Autodesk Inventor part; units mm, degrees
(part 2 of 2)
sketch "Sketch6" plane through (4.7625, 0, 0) normal (1, 0, 0) x (0, 0, -1)
  arc A0 (170.8837, 294.4565) -> (172.0866, 287.8113) centre (174.8077, 291.7353) ccw construction
  line L0 (170.8837, 294.4565) -> (172.7922, 297.2086) construction
  arc A1 (174.2704, 299.1942) -> (172.7922, 297.2086) centre (203.0571, 276.2209) ccw construction
  line L1 (174.2704, 299.1942) -> (186.7738, 314.8615) construction
  arc A2 (195.2416, 312.4978) -> (186.7738, 314.8615) centre (190.5061, 311.8829) ccw construction
  line L2 (195.2416, 312.4978) -> (195.6829, 309.0987) construction
  arc A3 (195.1019, 306.1294) -> (195.6829, 309.0987) centre (190.9475, 308.4838) ccw construction
  arc A4 (195.1019, 306.1294) -> (196.1286, 295.6536) centre (203.0571, 301.6209) ccw construction
  arc A5 (196.7071, 294.0954) -> (196.1286, 295.6536) centre (194.3195, 294.0954) ccw construction
  line L3 (196.7071, 294.0954) -> (196.7071, 292.4021) construction
  arc A6 (195.454, 290.3012) -> (196.7071, 292.4021) centre (194.3195, 292.4021) ccw construction
  arc A7 (195.454, 290.3012) -> (188.9768, 283.824) centre (203.0571, 276.2209) ccw construction
  arc A8 (186.8759, 282.5709) -> (188.9768, 283.824) centre (186.8759, 284.9585) ccw construction
  line L4 (186.8759, 282.5709) -> (186.0222, 282.5709) construction
  arc A9 (183.1524, 283.5294) -> (186.0222, 282.5709) centre (186.0222, 287.3461) ccw construction
  arc A10 (183.1524, 283.5294) -> (177.3062, 285.3581) centre (177.6571, 276.2209) ccw construction
  arc A11 (174.4018, 286.2058) -> (177.3062, 285.3581) centre (177.1229, 290.1298) ccw construction
  line L5 (174.4018, 286.2058) -> (172.0866, 287.8113) construction
  arc A12 (298.3468, 346.8044) -> (302.3019, 353.3428) centre (297.8735, 351.556) ccw construction
  line L6 (298.3468, 346.8044) -> (283.1869, 345.2944) construction
  arc A13 (278.6486, 347.5403) -> (283.1869, 345.2944) centre (282.7136, 350.046) ccw construction
  arc A14 (278.6486, 347.5403) -> (268.2318, 356.07) centre (261.0807, 336.7111) ccw construction
  arc A15 (265.1348, 360.076) -> (268.2318, 356.07) centre (269.8865, 360.5493) ccw construction
  line L7 (265.1348, 360.076) -> (263.6248, 375.236) construction
  arc A16 (269.2547, 380.403) -> (263.6248, 375.236) centre (268.3765, 375.7093) ccw construction
  arc A17 (302.3019, 353.3428) -> (269.2547, 380.403) centre (261.0807, 336.7111) ccw construction
  arc A18 (379.8681, 143.7131) -> (386.4173, 137.5565) centre (384.2479, 141.8105) ccw construction
  line L8 (379.8681, 143.7131) -> (390.24, 167.5887) construction
  arc A19 (394.413, 170.4568) -> (390.24, 167.5887) centre (394.6197, 165.686) ccw construction
  arc A20 (394.413, 170.4568) -> (413.0231, 184.3286) centre (393.5194, 191.0749) ccw construction
  arc A21 (416.9638, 187.5084) -> (413.0231, 184.3286) centre (417.536, 182.7676) ccw construction
  line L9 (416.9638, 187.5084) -> (432.089, 189.3339) construction
  arc A22 (437.3722, 183.813) -> (432.089, 189.3339) centre (432.6612, 184.5931) ccw construction
  arc A23 (413.7134, 151.4769) -> (437.3722, 183.813) centre (393.5194, 191.0749) ccw construction
  line L10 (413.7134, 151.4769) -> (386.4173, 137.5565) construction
  arc A24 (430.5672, 201.9424) -> (434.3852, 208.5618) centre (429.995, 206.6832) ccw construction
  line L11 (430.5672, 201.9424) -> (415.442, 200.1169) construction
  arc A25 (410.858, 202.2678) -> (415.442, 200.1169) centre (414.8698, 204.8577) ccw construction
  arc A26 (410.858, 202.2678) -> (400.2657, 210.5786) centre (393.5194, 191.0749) ccw construction
  arc A27 (397.0859, 214.5193) -> (400.2657, 210.5786) centre (401.8267, 215.0914) ccw construction
  line L12 (397.0859, 214.5193) -> (395.2604, 229.6445) construction
  arc A28 (400.7814, 234.9277) -> (395.2604, 229.6445) centre (400.0012, 230.2167) ccw construction
  arc A29 (434.3852, 208.5618) -> (400.7814, 234.9277) centre (393.5194, 191.0749) ccw construction
  arc A30 (250.9874, 373.9773) -> (244.449, 377.9323) centre (246.2357, 373.504) ccw construction
  line L13 (250.9874, 373.9773) -> (252.4974, 358.8173) construction
  arc A31 (250.2514, 354.2791) -> (252.4974, 358.8173) centre (247.7457, 358.344) ccw construction
  arc A32 (250.2514, 354.2791) -> (241.7218, 343.8623) centre (261.0807, 336.7111) ccw construction
  arc A33 (237.7157, 340.7653) -> (241.7218, 343.8623) centre (237.2424, 345.5169) ccw construction
  line L14 (237.7157, 340.7653) -> (216.1032, 338.6126) construction
  arc A34 (211.8976, 346.3429) -> (216.1032, 338.6126) centre (215.6299, 343.3643) ccw construction
  line L15 (211.8976, 346.3429) -> (226.3381, 364.4375) construction
  arc A35 (244.449, 377.9323) -> (226.3381, 364.4375) centre (261.0807, 336.7111) ccw construction
  arc A36 (198.999, 204.1865) -> (205.9543, 209.4304) centre (201.2979, 208.3719) ccw construction
  line L16 (198.999, 204.1865) -> (188.5021, 209.9521) construction
  arc A37 (186.0315, 214.3721) -> (188.5021, 209.9521) centre (190.801, 214.1375) ccw construction
  arc A38 (186.0315, 214.3721) -> (185.1217, 221.5267) centre (165.4189, 215.3861) ccw construction
  arc A39 (186.4073, 226.4244) -> (185.1217, 221.5267) centre (189.6806, 222.9476) ccw construction
  line L17 (186.4073, 226.4244) -> (193.2473, 232.864) construction
  arc A40 (201.177, 230.4457) -> (193.2473, 232.864) centre (196.5206, 229.3871) ccw construction
  line L18 (201.177, 230.4457) -> (205.9543, 209.4304) construction
  arc A41 (211.3352, 325.3748) -> (207.073, 320.0083) centre (211.8085, 320.6231) ccw construction
  line L19 (211.3352, 325.3748) -> (238.9744, 328.1278) construction
  arc A42 (243.5127, 325.8818) -> (238.9744, 328.1278) centre (239.4477, 323.3761) ccw construction
  arc A43 (243.5127, 325.8818) -> (244.321, 324.6686) centre (261.0807, 336.7111) ccw construction
  arc A44 (244.646, 319.6154) -> (244.321, 324.6686) centre (240.4431, 321.8822) ccw construction
  line L20 (244.646, 319.6154) -> (226.8389, 286.5977) construction
  arc A45 (224.633, 284.5268) -> (226.8389, 286.5977) centre (222.636, 288.8644) ccw construction
  arc A46 (224.633, 284.5268) -> (222.4898, 283.1494) centre (228.4571, 276.2209) ccw construction
  arc A47 (220.9317, 282.5709) -> (222.4898, 283.1494) centre (220.9317, 284.9585) ccw construction
  line L21 (220.9317, 282.5709) -> (219.2384, 282.5709) construction
  arc A48 (217.1375, 283.824) -> (219.2384, 282.5709) centre (219.2384, 284.9585) ccw construction
  arc A49 (217.1375, 283.824) -> (210.6603, 290.3012) centre (203.0571, 276.2209) ccw construction
  arc A50 (209.4071, 292.4021) -> (210.6603, 290.3012) centre (211.7947, 292.4021) ccw construction
  line L22 (209.4071, 292.4021) -> (209.4071, 294.0954) construction
  arc A51 (209.9856, 295.6536) -> (209.4071, 294.0954) centre (211.7947, 294.0954) ccw construction
  arc A52 (209.9856, 295.6536) -> (209.5973, 308.0115) centre (203.0571, 301.6209) ccw construction
  arc A53 (208.2772, 310.7339) -> (209.5973, 308.0115) centre (213.0127, 311.3488) ccw construction
  line L23 (208.2772, 310.7339) -> (207.073, 320.0083) construction
  arc A54 (219.2384, 269.8709) -> (217.1375, 268.6177) centre (219.2384, 267.4833) ccw construction
  line L24 (219.2384, 269.8709) -> (220.9317, 269.8709) construction
  arc A55 (222.4898, 269.2924) -> (220.9317, 269.8709) centre (220.9317, 267.4833) ccw construction
  arc A56 (222.4898, 269.2924) -> (232.2342, 267.8934) centre (228.4571, 276.2209) ccw construction
  arc A57 (235.2436, 268.2059) -> (232.2342, 267.8934) centre (234.2067, 263.5446) ccw construction
  line L25 (235.2436, 268.2059) -> (318.0387, 249.787) construction
  arc A58 (321.7764, 245.0563) -> (318.0387, 249.787) centre (317.0017, 245.1258) ccw construction
  line L26 (321.7764, 245.0563) -> (320.5418, 160.2462) construction
  arc A59 (319.5416, 157.3907) -> (320.5418, 160.2462) centre (315.7671, 160.3157) ccw construction
  arc A60 (319.5416, 157.3907) -> (317.8734, 149.6741) centre (326.7693, 151.7896) ccw construction
  arc A61 (317.6048, 146.6604) -> (317.8734, 149.6741) centre (313.2278, 148.5693) ccw construction
  line L27 (317.6048, 146.6604) -> (317.2174, 145.7719) construction
  arc A62 (315.236, 144.3478) -> (317.2174, 145.7719) centre (315.0288, 146.7264) ccw construction
  arc A63 (315.236, 144.3478) -> (306.8489, 141.0546) centre (316.6157, 128.5073) ccw construction
  arc A64 (304.4279, 140.7502) -> (306.8489, 141.0546) centre (305.3824, 142.9387) ccw construction
  line L28 (304.4279, 140.7502) -> (302.7698, 141.4733) construction
  arc A65 (301.5729, 142.6264) -> (302.7698, 141.4733) centre (303.7243, 143.6618) ccw construction
  arc A66 (301.5729, 142.6264) -> (291.2986, 147.5757) centre (293.3334, 138.661) ccw construction
  arc A67 (288.2875, 147.8716) -> (291.2986, 147.5757) centre (290.2359, 152.2312) ccw construction
  line L29 (288.2875, 147.8716) -> (248.8959, 165.4772) construction
  arc A68 (246.7674, 167.3507) -> (248.8959, 165.4772) centre (250.8444, 169.8368) ccw construction
  arc A69 (246.7674, 167.3507) -> (245.8371, 168.6073) centre (239.3128, 162.8049) ccw construction
  arc A70 (244.6507, 171.3375) -> (245.8371, 168.6073) centre (249.4053, 171.7808) ccw construction
  arc A71 (244.6507, 171.3375) -> (242.4292, 176.382) centre (235.9761, 170.5287) ccw construction
  line L30 (242.4292, 176.382) -> (231.9513, 187.9335) construction
  arc A72 (231.9513, 187.9335) -> (227.1533, 190.6337) centre (225.4982, 182.0802) ccw construction
  arc A73 (224.5561, 192.0782) -> (227.1533, 190.6337) centre (228.0605, 195.3219) ccw construction
  arc A74 (224.5561, 192.0782) -> (223.7494, 192.8453) centre (218.1439, 186.1428) ccw construction
  arc A75 (222.1565, 195.4498) -> (223.7494, 192.8453) centre (226.8129, 196.5083) ccw construction
  line L31 (222.1565, 195.4498) -> (211.1035, 244.0716) construction
  arc A76 (211.402, 247.0824) -> (211.1035, 244.0716) centre (215.7599, 245.1301) ccw construction
  arc A77 (211.402, 247.0824) -> (209.9856, 256.7882) centre (203.0571, 250.8209) ccw construction
  arc A78 (209.4071, 258.3463) -> (209.9856, 256.7882) centre (211.7947, 258.3463) ccw construction
  line L32 (209.4071, 258.3463) -> (209.4071, 260.0397) construction
  arc A79 (210.6603, 262.1405) -> (209.4071, 260.0397) centre (211.7947, 260.0397) ccw construction
  arc A80 (210.6603, 262.1405) -> (217.1375, 268.6177) centre (203.0571, 276.2209) ccw construction
  arc A81 (337.1993, 150.5599) -> (335.2123, 148.2783) centre (339.6214, 146.4446) ccw construction
  line L33 (337.1993, 150.5599) -> (367.2672, 168.2562) construction
  arc A82 (374.069, 162.2382) -> (367.2672, 168.2562) centre (369.6893, 164.1408) ccw construction
  line L34 (374.069, 162.2382) -> (363.4789, 137.8602) construction
  arc A83 (361.2833, 135.5164) -> (363.4789, 137.8602) centre (359.0991, 139.7628) ccw construction
  arc A84 (361.2833, 135.5164) -> (357.5507, 132.0949) centre (365.675, 126.9785) ccw construction
  arc A85 (355.0252, 130.1112) -> (357.5507, 132.0949) centre (353.51, 134.6396) ccw construction
  line L35 (355.0252, 130.1112) -> (345.8158, 127.0298) construction
  arc A86 (342.7902, 127.0282) -> (345.8158, 127.0298) centre (344.3006, 131.5582) ccw construction
  arc A87 (342.7902, 127.0282) -> (337.1978, 127.0899) centre (339.8979, 118.3537) ccw construction
  arc A88 (335.5383, 127.1825) -> (337.1978, 127.0899) centre (336.4928, 129.3711) ccw construction
  line L36 (335.5383, 127.1825) -> (335.1284, 127.3613) construction
  arc A89 (332.3207, 130.9922) -> (335.1284, 127.3613) centre (337.0372, 131.7384) ccw construction
  arc A90 (332.3207, 130.9922) -> (329.1629, 138.2741) centre (316.6157, 128.5073) ccw construction
  arc A91 (328.8585, 140.6951) -> (329.1629, 138.2741) centre (331.047, 139.7406) ccw construction
  line L37 (328.8585, 140.6951) -> (329.246, 141.5836) construction
  arc A92 (331.2718, 143.8309) -> (329.246, 141.5836) centre (333.623, 139.6747) ccw construction
  arc A93 (331.2718, 143.8309) -> (335.2123, 148.2783) centre (326.7693, 151.7896) ccw construction
  arc A94 (382.3265, 208.4134) -> (384.4774, 212.9975) centre (379.7366, 212.4253) ccw construction
  arc A95 (382.3265, 208.4134) -> (372.946, 189.4499) centre (393.5194, 191.0749) ccw construction
  arc A96 (370.6077, 184.9585) -> (372.946, 189.4499) centre (368.1856, 189.0739) ccw construction
  line L38 (370.6077, 184.9585) -> (340.6035, 167.2997) construction
  arc A97 (333.4067, 171.4846) -> (340.6035, 167.2997) centre (338.1814, 171.4151) ccw construction
  line L39 (333.4067, 171.4846) -> (334.4104, 240.4277) construction
  arc A98 (341.5331, 244.5162) -> (334.4104, 240.4277) centre (339.1851, 240.3582) ccw construction
  arc A99 (341.5331, 244.5162) -> (377.7123, 234.6667) centre (379.0508, 310.9542) ccw construction
  arc A100 (382.3693, 230.4644) -> (377.7123, 234.6667) centre (377.6285, 229.8922) ccw construction
  line L40 (382.3693, 230.4644) -> (384.4774, 212.9975) construction
  arc A101 (241.0284, 286.1531) -> (244.1944, 279.2252) centre (245.2313, 283.8864) ccw construction
  line L41 (241.0284, 286.1531) -> (255.824, 313.5869) construction
  arc A102 (260.2249, 316.0913) -> (255.824, 313.5869) centre (260.0269, 311.3202) ccw construction
  arc A103 (260.2249, 316.0913) -> (280.4395, 329.5599) centre (261.0807, 336.7111) ccw construction
  arc A104 (284.4456, 332.6569) -> (280.4395, 329.5599) centre (284.9189, 327.9052) ccw construction
  line L42 (284.4456, 332.6569) -> (299.6056, 334.1669) construction
  arc A105 (304.7726, 328.5371) -> (299.6056, 334.1669) centre (300.0789, 329.4152) ccw construction
  arc A106 (304.5076, 327.2295) -> (304.7726, 328.5371) centre (261.0807, 336.7111) ccw construction
  arc A107 (304.5076, 327.2295) -> (313.4045, 272.0681) centre (379.0508, 310.9542) ccw construction
  arc A108 (308.259, 264.9731) -> (313.4045, 272.0681) centre (309.296, 269.6344) ccw construction
  line L43 (308.259, 264.9731) -> (244.1944, 279.2252) construction
  arc A109 (185.1826, 269.8709) -> (183.6244, 269.2924) centre (185.1826, 267.4833) ccw construction
  line L44 (185.1826, 269.8709) -> (185.5094, 269.8709) construction
  arc A110 (189.5424, 267.6526) -> (185.5094, 269.8709) centre (185.5094, 265.0957) ccw construction
  arc A111 (189.5424, 267.6526) -> (195.454, 262.1405) centre (203.0571, 276.2209) ccw construction
  arc A112 (196.7071, 260.0397) -> (195.454, 262.1405) centre (194.3195, 260.0397) ccw construction
  line L45 (196.7071, 260.0397) -> (196.7071, 259.1859) construction
  arc A113 (195.7486, 256.3162) -> (196.7071, 259.1859) centre (191.9319, 259.1859) ccw construction
  arc A114 (195.7486, 256.3162) -> (194.0462, 252.3753) centre (203.0571, 250.8209) ccw construction
  arc A115 (192.6138, 249.7103) -> (194.0462, 252.3753) centre (189.3405, 253.1871) ccw construction
  line L46 (192.6138, 249.7103) -> (177.7018, 235.6713) construction
  arc A116 (172.7356, 234.683) -> (177.7018, 235.6713) centre (174.4285, 239.1481) ccw construction
  arc A117 (172.7356, 234.683) -> (164.402, 235.9985) centre (165.4189, 215.3861) ccw construction
  arc A118 (159.9817, 238.4684) -> (164.402, 235.9985) centre (164.1668, 240.7679) ccw construction
  line L47 (159.9817, 238.4684) -> (154.2435, 248.9118) construction
  arc A119 (155.9126, 255.2699) -> (154.2435, 248.9118) centre (158.4286, 251.2113) ccw construction
  line L48 (155.9126, 255.2699) -> (173.8931, 266.4164) construction
  arc A120 (176.8373, 267.1137) -> (173.8931, 266.4164) centre (176.4091, 262.3577) ccw construction
  arc A121 (176.8373, 267.1137) -> (183.6244, 269.2924) centre (177.6571, 276.2209) ccw construction
  circle A122 centre (62.0508, 103.0707) radius 3.2512 construction
  circle A123 centre (365.675, 126.9785) radius 3.2512 construction
  circle A124 centre (116.952, 9.0853) radius 3.2512 construction
  circle A125 centre (143.5951, 255.1053) radius 3.2512 construction
  circle A126 centre (199.3, 330.5575) radius 3.2512 construction
  circle A127 centre (219.5153, 55.5753) radius 3.2512 construction
  line L49 (167.5741, 300.8271) -> (63.5783, 150.8617) construction
  arc A128 (63.5783, 150.8617) -> (59.1713, 138.8602) centre (84.4507, 136.3874) ccw construction
  line L50 (59.1713, 138.8602) -> (51.0413, 55.7455) construction
  arc A129 (51.0413, 55.7455) -> (122.6227, 4.5541) centre (101.6, 50.8) ccw construction
  line L51 (122.6227, 4.5541) -> (278.1353, 75.2478) construction
  arc A130 (278.1353, 75.2478) -> (279.5746, 75.9415) centre (263.4194, 107.6199) ccw construction
  line L52 (279.5746, 75.9415) -> (416.5983, 145.82) construction
  arc A131 (416.5983, 145.82) -> (387.4324, 241.5089) centre (393.5194, 191.0749) ccw construction
  arc A132 (310.7115, 325.875) -> (387.4324, 241.5089) centre (379.0508, 310.9542) ccw construction
  arc A133 (310.7115, 325.875) -> (221.3748, 368.3984) centre (261.0807, 336.7111) ccw construction
  line L53 (221.3748, 368.3984) -> (169.3072, 303.1551) construction
  arc A134 (169.3072, 303.1551) -> (167.5741, 300.8271) centre (203.0571, 276.2209) ccw construction
  circle A135 centre (326.7693, 151.7896) radius 2.794 construction
  circle A136 centre (172.549, 123.5241) radius 3.2512 construction
  circle A137 centre (203.0571, 276.2209) radius 9.652 construction
  circle A138 centre (228.4571, 276.2209) radius 2.794 construction
  circle A139 centre (203.0571, 250.8209) radius 2.794 construction
  circle A140 centre (177.6571, 276.2209) radius 2.794 construction
  circle A141 centre (84.4507, 136.3874) radius 14.2875 construction
  circle A142 centre (263.4194, 107.6199) radius 14.2875 construction
  circle A143 centre (316.6157, 128.5073) radius 9.5504 construction
  circle A144 centre (239.3128, 162.8049) radius 2.3812 construction
  circle A145 centre (218.1439, 186.1428) radius 2.3876 construction
  arc A146 (219.8851, 180.1779) -> (219.7225, 176.8412) centre (221.4722, 178.4283) ccw construction
  line L54 (219.8851, 180.1779) -> (223.9112, 183.8298) construction
  arc A147 (227.2479, 183.6672) -> (223.9112, 183.8298) centre (225.4982, 182.0802) ccw construction
  line L55 (227.2479, 183.6672) -> (237.7258, 172.1157) construction
  arc A148 (237.5632, 168.779) -> (237.7258, 172.1157) centre (235.9761, 170.5287) ccw construction
  line L56 (237.5632, 168.779) -> (233.5371, 165.1271) construction
  arc A149 (230.2004, 165.2897) -> (233.5371, 165.1271) centre (231.9501, 166.8768) ccw construction
  line L57 (230.2004, 165.2897) -> (219.7225, 176.8412) construction
  circle A150 centre (339.8979, 118.3537) radius 2.794 construction
  circle A151 centre (306.462, 105.2251) radius 2.794 construction
  circle A152 centre (293.3334, 138.661) radius 2.794 construction
  circle A153 centre (103.7307, 197.6195) radius 3.2512 construction
  circle A154 centre (203.0571, 301.6209) radius 2.794 construction
  circle A155 centre (101.6, 50.8) radius 14.2875 construction
  circle A156 centre (165.4189, 215.3861) radius 14.2875 construction
  circle A157 centre (393.5194, 191.0749) radius 14.2875 construction
  circle A158 centre (261.0807, 336.7111) radius 14.2875 construction
  line L58 (68.7964, 147.2431) -> (172.7922, 297.2086) construction
  arc A159 (174.2704, 299.1942) -> (172.7922, 297.2086) centre (203.0571, 276.2209) ccw construction
  line L59 (174.2704, 299.1942) -> (226.3381, 364.4375) construction
  arc A160 (304.5076, 327.2295) -> (226.3381, 364.4375) centre (261.0807, 336.7111) ccw construction
  arc A161 (304.5076, 327.2295) -> (388.1933, 235.2047) centre (379.0508, 310.9542) ccw construction
  arc A162 (413.7134, 151.4769) -> (388.1933, 235.2047) centre (393.5194, 191.0749) ccw construction
  line L60 (413.7134, 151.4769) -> (276.6898, 81.5983) construction
  arc A163 (275.5075, 81.0285) -> (276.6898, 81.5983) centre (263.4194, 107.6199) ccw construction
  line L61 (275.5075, 81.0285) -> (119.9949, 10.3348) construction
  arc A164 (57.3611, 55.1273) -> (119.9949, 10.3348) centre (101.6, 50.8) ccw construction
  line L62 (57.3611, 55.1273) -> (65.4912, 138.242) construction
  arc A165 (68.7964, 147.2431) -> (65.4912, 138.242) centre (84.4507, 136.3874) ccw construction
  circle A166 centre (143.5951, 255.1053) radius 9.6012 construction
  circle A167 centre (165.4189, 215.3861) radius 20.6375 construction
  circle A168 centre (103.7307, 197.6195) radius 9.6012 construction
  circle A169 centre (172.549, 123.5241) radius 9.6012 construction
  circle A170 centre (84.4507, 136.3874) radius 20.6375 construction
  circle A171 centre (62.0508, 103.0707) radius 9.6012 construction
  circle A172 centre (218.1439, 186.1428) radius 8.7376 construction
  arc A173 (215.6189, 184.8813) -> (215.0191, 172.575) centre (221.4722, 178.4283) ccw construction
  line L63 (215.6189, 184.8813) -> (219.6449, 188.5332) construction
  arc A174 (231.9513, 187.9335) -> (219.6449, 188.5332) centre (225.4982, 182.0802) ccw construction
  line L64 (231.9513, 187.9335) -> (242.4292, 176.382) construction
  arc A175 (241.8294, 164.0757) -> (242.4292, 176.382) centre (235.9761, 170.5287) ccw construction
  line L65 (241.8294, 164.0757) -> (237.8033, 160.4238) construction
  arc A176 (225.497, 161.0235) -> (237.8033, 160.4238) centre (231.9501, 166.8768) ccw construction
  line L66 (225.497, 161.0235) -> (215.0191, 172.575) construction
  circle A177 centre (239.3128, 162.8049) radius 8.7312 construction
  circle A178 centre (293.3334, 138.661) radius 9.144 construction
  circle A179 centre (316.6157, 128.5073) radius 15.9004 construction
  circle A180 centre (306.462, 105.2251) radius 9.144 construction
  circle A181 centre (263.4194, 107.6199) radius 20.6375 construction
  circle A182 centre (219.5153, 55.5753) radius 9.6012 construction
  circle A183 centre (101.6, 50.8) radius 20.6375 construction
  circle A184 centre (116.952, 9.0853) radius 9.6012 construction
  line L67 (145.5875, 209.6745) -> (112.9569, 200.2767) construction
  line L68 (148.2185, 246.6906) -> (155.4809, 233.4731) construction
  line L69 (167.016, 194.8105) -> (171.806, 133.0965) construction
  line L70 (100.8472, 188.4616) -> (90.6488, 156.0722) construction
  line L71 (104.8717, 133.4057) -> (163.0486, 124.9113) construction
  line L72 (183.4664, 205.3763) -> (210.5028, 190.3808) construction
  line L73 (179.6605, 129.9747) -> (220.2581, 166.7992) construction
  line L74 (242.808, 154.8037) -> (255.1581, 126.5317) construction
  line L75 (247.2842, 159.2422) -> (284.9853, 142.3921) construction
  line L76 (286.9883, 132.0768) -> (277.7401, 122.4801) construction
  line L77 (284.0251, 106.4735) -> (297.3321, 105.7331) construction
  line L78 (310.2595, 113.9327) -> (310.1173, 113.6067) construction
  line L79 (301.715, 135.0057) -> (302.041, 134.8635) construction
  line L80 (250.1124, 91.8456) -> (225.7061, 62.914) construction
  line L81 (243.091, 111.1778) -> (182.0065, 121.8689) construction
  line L82 (178.0082, 115.626) -> (214.0561, 63.4734) construction
  line L83 (165.8443, 116.6517) -> (116.0115, 65.5721) construction
  line L84 (122.2206, 51.6351) -> (209.922, 55.1868) construction
  line L85 (108.7277, 31.4324) -> (113.6359, 18.0956) construction
  line L86 (87.1885, 36.0279) -> (70.5598, 18.9832) construction
  line L87 (88.5053, 116.1521) -> (97.5454, 71.0353) construction
  line L88 (67.8439, 95.4142) -> (89.1479, 67.2575) construction
  line L89 (72.936, 119.2609) -> (67.4078, 111.0385) construction
  line L90 (142.4146, 244.0672) -> (148.8512, 232.3527)
  line L91 (141.7059, 215.1647) -> (122.3457, 209.5888)
  arc A185 (139.8047, 246.284) -> (140.0117, 246.1979) centre (143.5951, 255.1053) ccw
  arc A186 (148.5657, 227.2972) -> (145.0885, 218.9327) centre (165.4189, 215.3861) ccw
  line L92 (117.1001, 216.8987) -> (136.9001, 245.4509)
  arc A187 (148.5657, 227.2972) -> (148.8512, 232.3527) centre (144.6661, 230.0532) ccw
  arc A188 (141.7059, 215.1647) -> (145.0885, 218.9327) centre (140.3843, 219.7534) ccw
  arc A189 (142.4146, 244.0672) -> (140.0117, 246.1979) centre (138.2295, 241.7677) ccw
  arc A190 (117.1001, 216.8987) -> (122.3457, 209.5888) centre (121.0241, 214.1775) ccw
  circle A191 centre (138.8621, 244.0903) radius 2.3876 construction
  arc A192 (139.8047, 246.284) -> (136.9001, 245.4509) centre (138.8621, 244.0903) ccw
  line L93 (145.2207, 202.9608) -> (114.238, 194.0376)
  line L94 (107.0529, 187.0272) -> (97.3696, 156.2736)
  line L95 (107.9765, 139.3697) -> (159.6899, 131.819)
  line L96 (160.8561, 192.1151) -> (165.1407, 136.9136)
  arc A193 (104.1161, 142.6465) -> (98.6409, 151.3722) centre (84.4507, 136.3874) ccw
  arc A194 (150.0893, 201.5691) -> (157.8472, 196.1878) centre (165.4189, 215.3861) ccw
  arc A195 (108.9913, 189.5877) -> (111.6305, 192.1628) centre (103.7307, 197.6195) ccw
  arc A196 (97.3696, 156.2736) -> (98.6409, 151.3722) centre (101.9243, 154.8395) ccw
  arc A197 (104.1161, 142.6465) -> (107.9765, 139.3697) centre (108.6664, 144.0948) ccw
  arc A198 (159.6899, 131.819) -> (165.1407, 136.9136) centre (160.3798, 136.5441) ccw
  arc A199 (150.0893, 201.5691) -> (145.2207, 202.9608) centre (146.5423, 198.3721) ccw
  arc A200 (160.8561, 192.1151) -> (157.8472, 196.1878) centre (156.0952, 191.7456) ccw
  arc A201 (114.238, 194.0376) -> (111.6305, 192.1628) centre (115.5595, 189.4489) ccw
  arc A202 (108.9913, 189.5877) -> (107.0529, 187.0272) centre (111.6076, 185.5931) ccw
  line L97 (182.3196, 198.751) -> (208.3567, 184.3098)
  line L98 (173.518, 193.0979) -> (177.1237, 146.6426)
  line L99 (185.0928, 143.4752) -> (212.7408, 168.5537)
  arc A203 (175.8624, 197.5861) -> (177.263, 198.4856) centre (165.4189, 215.3861) ccw
  arc A204 (210.3177, 182.2574) -> (211.6131, 180.3381) centre (218.1439, 186.1428) ccw
  arc A205 (212.7982, 177.6127) -> (213.775, 174.2825) centre (221.8723, 178.4659) ccw
  arc A206 (177.1237, 146.6426) -> (185.0928, 143.4752) centre (181.8846, 147.0122) ccw
  arc A207 (182.3196, 198.751) -> (177.263, 198.4856) centre (180.0035, 194.5751) ccw
  arc A208 (175.8624, 197.5861) -> (173.518, 193.0979) centre (178.2789, 193.4674) ccw
  arc A209 (212.7408, 168.5537) -> (213.775, 174.2825) centre (209.5326, 172.0906) ccw
  arc A210 (212.7982, 177.6127) -> (211.6131, 180.3381) centre (208.044, 177.1657) ccw
  arc A211 (210.3177, 182.2574) -> (208.3567, 184.3098) centre (206.0406, 180.1339) ccw
  line L100 (193.6591, 134.0992) -> (221.2962, 159.1677)
  line L101 (236.5596, 153.2447) -> (248.4542, 126.0155)
  line L102 (242.0082, 117.8138) -> (196.0441, 125.8585)
  arc A212 (247.7126, 121.0065) -> (246.7001, 119.7182) centre (263.4194, 107.6199) ccw
  arc A213 (232.9035, 156.8757) -> (234.7042, 155.389) centre (239.3128, 162.8049) ccw
  arc A214 (227.1405, 159.6124) -> (230.3016, 158.322) centre (231.9501, 166.8768) ccw
  line L103 (224.5243, 162.0959) -> (225.497, 161.0235)
  arc A215 (193.6591, 134.0992) -> (196.0441, 125.8585) centre (196.8673, 130.5622) ccw
  arc A216 (247.7126, 121.0065) -> (248.4542, 126.0155) centre (244.0783, 124.104) ccw
  arc A217 (242.0082, 117.8138) -> (246.7001, 119.7182) centre (242.8314, 122.5175) ccw
  arc A218 (227.1405, 159.6124) -> (221.2962, 159.1677) centre (224.5044, 155.6308) ccw
  arc A219 (232.9035, 156.8757) -> (230.3016, 158.322) centre (229.3981, 153.633) ccw
  arc A220 (236.5596, 153.2447) -> (234.7042, 155.389) centre (232.1837, 151.3332) ccw
  line L104 (303.8285, 115.0715) -> (303.9854, 115.4311)
  line L105 (297.693, 129.8322) -> (298.103, 129.6534)
  line L106 (292.1012, 128.2313) -> (284.8365, 120.693)
  line L107 (288.0097, 112.6116) -> (298.4626, 112.03)
  arc A221 (283.3782, 112.8693) -> (281.6177, 117.3529) centre (263.4194, 107.6199) ccw
  arc A222 (301.9596, 113.1838) -> (301.3812, 112.8276) centre (306.462, 105.2251) ccw
  arc A223 (294.7827, 129.6326) -> (296.0335, 129.9248) centre (293.3334, 138.661) ccw
  arc A224 (300.9106, 126.0225) -> (303.4157, 119.6426) centre (316.6157, 128.5073) ccw
  arc A225 (300.9106, 126.0225) -> (298.103, 129.6534) centre (296.1941, 125.2763) ccw
  arc A226 (303.8285, 115.0715) -> (303.4157, 119.6426) centre (299.4515, 116.9804) ccw
  arc A227 (301.9596, 113.1838) -> (303.9854, 115.4311) centre (299.6083, 117.34) ccw
  arc A228 (298.4626, 112.03) -> (301.3812, 112.8276) centre (298.7279, 116.7978) ccw
  arc A229 (284.8365, 120.693) -> (288.0097, 112.6116) centre (288.275, 117.3794) ccw
  arc A230 (294.7827, 129.6326) -> (292.1012, 128.2313) centre (295.5396, 124.9178) ccw
  circle A231 centre (296.7386, 127.6436) radius 2.3876 construction
  arc A232 (297.693, 129.8322) -> (296.0335, 129.9248) centre (296.7386, 127.6436) ccw
  line L108 (262.9615, 145.28) -> (276.2747, 139.3298)
  line L109 (277.7647, 131.6567) -> (274.7017, 128.4782)
  line L110 (256.6371, 139.0089) -> (260.0922, 131.0994)
  arc A233 (269.7893, 127.2498) -> (264.2711, 128.2398) centre (263.4194, 107.6199) ccw
  arc A234 (262.9615, 145.28) -> (256.6371, 139.0089) centre (261.013, 140.9204) ccw
  arc A235 (277.7647, 131.6567) -> (276.2747, 139.3298) centre (274.3263, 134.9702) ccw
  arc A236 (269.7893, 127.2498) -> (274.7017, 128.4782) centre (271.2632, 131.7918) ccw
  arc A237 (260.0922, 131.0994) -> (264.2711, 128.2398) centre (264.4682, 133.011) ccw
  line L111 (285.8795, 100.0105) -> (292.479, 99.6433)
  line L112 (253.5407, 86.0614) -> (246.6512, 77.8946)
  line L113 (252.2773, 70.4684) -> (275.5075, 81.0285)
  line L114 (294.3831, 90.6215) -> (276.6898, 81.5983)
  arc A238 (275.5075, 81.0285) -> (276.6898, 81.5983) centre (263.4194, 107.6199) ccw
  arc A239 (258.3611, 87.6119) -> (281.4437, 97.5684) centre (263.4194, 107.6199) ccw
  arc A240 (258.3611, 87.6119) -> (253.5407, 86.0614) centre (257.1906, 82.9824) ccw
  arc A241 (246.6512, 77.8946) -> (252.2773, 70.4684) centre (250.3012, 74.8155) ccw
  arc A242 (285.8795, 100.0105) -> (281.4437, 97.5684) centre (285.6142, 95.2426) ccw
  arc A243 (299.5399, 99.2504) -> (305.2476, 96.1621) centre (306.462, 105.2251) ccw
  arc A244 (294.3831, 90.6215) -> (292.479, 99.6433) centre (292.2137, 94.8754) ccw
  line L115 (239.8187, 105.304) -> (197.6387, 112.6864)
  line L116 (192.8872, 105.2675) -> (216.4656, 71.1553)
  line L117 (243.8334, 94.2504) -> (224.0438, 70.7914)
  arc A245 (243.5849, 101.9193) -> (244.5496, 99.2631) centre (263.4194, 107.6199) ccw
  arc A246 (197.6387, 112.6864) -> (192.8872, 105.2675) centre (196.8154, 107.9827) ccw
  arc A247 (243.5849, 101.9193) -> (239.8187, 105.304) centre (238.9955, 100.6003) ccw
  arc A248 (243.8334, 94.2504) -> (244.5496, 99.2631) centre (240.1835, 97.3294) ccw
  arc A249 (216.4656, 71.1553) -> (224.0438, 70.7914) centre (220.3938, 73.8705) ccw
  line L118 (106.1416, 126.803) -> (150.0332, 120.3943)
  line L119 (95.1658, 115.2322) -> (103.3374, 74.4504)
  line L120 (152.7613, 112.3346) -> (113.01, 71.5887)
  arc A250 (96.9547, 119.9692) -> (101.5055, 124.7667) centre (84.4507, 136.3874) ccw
  arc A251 (108.0902, 70.3904) -> (106.8132, 70.7682) centre (101.6, 50.8) ccw
  arc A252 (106.1416, 126.803) -> (101.5055, 124.7667) centre (105.4517, 122.0779) ccw
  arc A253 (96.9547, 119.9692) -> (95.1658, 115.2322) centre (99.848, 116.1703) ccw
  arc A254 (152.7613, 112.3346) -> (150.0332, 120.3943) centre (149.3433, 115.6692) ccw
  arc A255 (108.0902, 70.3904) -> (113.01, 71.5887) centre (109.5919, 74.9233) ccw
  arc A256 (103.3374, 74.4504) -> (106.8132, 70.7682) centre (108.0195, 75.3885) ccw
  line L121 (167.6605, 109.42) -> (125.6733, 66.3823)
  line L122 (175.0067, 108.8006) -> (202.8011, 68.5888)
  line L123 (129.2845, 58.2764) -> (199.0662, 61.1024)
  arc A257 (175.0067, 108.8006) -> (167.6605, 109.42) centre (171.0785, 106.0854) ccw
  arc A258 (199.0662, 61.1024) -> (202.8011, 68.5888) centre (198.8729, 65.8737) ccw
  arc A259 (125.6733, 66.3823) -> (129.2845, 58.2764) centre (129.0913, 63.0477) ccw
  line L124 (115.4504, 31.551) -> (119.7664, 19.8236)
  line L125 (124.6863, 45.3797) -> (179.7658, 47.6103)
  line L126 (129.3853, 14.6036) -> (181.9351, 38.4919)
  arc A260 (116.4871, 36.5074) -> (120.5052, 42.5235) centre (101.6, 50.8) ccw
  arc A261 (124.6863, 45.3797) -> (120.5052, 42.5235) centre (124.8796, 40.6084) ccw
  arc A262 (116.4871, 36.5074) -> (115.4504, 31.551) centre (119.9318, 33.2003) ccw
  arc A263 (123.9358, 15.6738) -> (121.8244, 17.3583) centre (116.952, 9.0853) ccw
  arc A264 (119.7664, 19.8236) -> (121.8244, 17.3583) centre (124.2477, 21.4729) ccw
  arc A265 (123.9358, 15.6738) -> (129.3853, 14.6036) centre (127.4092, 18.9507) ccw
  arc A266 (181.9351, 38.4919) -> (179.7658, 47.6103) centre (179.959, 42.839) ccw
  line L127 (103.5319, 27.1647) -> (107.8479, 15.4373)
  line L128 (90.19, 30.0113) -> (79.5512, 19.1063)
  arc A267 (95.1098, 31.2096) -> (99.5296, 30.2666) centre (101.6, 50.8) ccw
  arc A268 (80.7269, 11.5557) -> (102.8585, 6.3678) centre (101.6, 50.8) ccw
  arc A269 (107.879, 12.226) -> (107.4494, 10.4582) centre (116.952, 9.0853) ccw
  arc A270 (95.1098, 31.2096) -> (90.19, 30.0113) centre (93.6081, 26.6767) ccw
  arc A271 (103.5319, 27.1647) -> (99.5296, 30.2666) centre (99.0506, 25.5155) ccw
  arc A272 (107.879, 12.226) -> (107.8479, 15.4373) centre (103.3665, 13.7881) ccw
  arc A273 (102.8585, 6.3678) -> (107.4494, 10.4582) centre (102.7233, 11.1411) ccw
  arc A274 (79.5512, 19.1063) -> (80.7269, 11.5557) centre (82.9692, 15.7717) ccw
  line L129 (83.4696, 108.9629) -> (85.8233, 97.2162)
  line L130 (74.8246, 110.689) -> (72.401, 107.0842)
  line L131 (72.6087, 99.6409) -> (77.3331, 93.3968)
  arc A275 (83.4696, 108.9629) -> (74.8246, 110.689) centre (78.7874, 108.0247) ccw
  arc A276 (71.645, 102.7043) -> (71.6097, 103.9717) centre (62.0508, 103.0707) ccw
  arc A277 (72.401, 107.0842) -> (71.6097, 103.9717) centre (76.3638, 104.4199) ccw
  arc A278 (71.645, 102.7043) -> (72.6087, 99.6409) centre (76.4168, 102.5221) ccw
  arc A279 (77.3331, 93.3968) -> (85.8233, 97.2162) centre (81.1411, 96.278) ccw
  line L132 (68.5105, 84.0091) -> (82.7502, 65.189)
  line L133 (81.0995, 38.8799) -> (70.4607, 27.9749)
  line L134 (59.9499, 81.5928) -> (57.3611, 55.1273)
  arc A280 (57.3611, 55.1273) -> (62.8834, 28.9637) centre (101.6, 50.8) ccw
  arc A281 (83.1997, 60.1454) -> (82.1759, 43.8278) centre (101.6, 50.8) ccw
  arc A282 (68.5105, 84.0091) -> (59.9499, 81.5928) centre (64.7024, 81.1279) ccw
  arc A283 (83.1997, 60.1454) -> (82.7502, 65.189) centre (78.9422, 62.3077) ccw
  arc A284 (81.0995, 38.8799) -> (82.1759, 43.8278) centre (77.6815, 42.2145) ccw
  arc A285 (62.8834, 28.9637) -> (70.4607, 27.9749) centre (67.0427, 31.3095) ccw
  point P0 (0, 0)
  point P1 (224.9615, 171.0655)
  point P2 (141.4977, 245.736)
  point P3 (150.3978, 229.5378)
  point P4 (109.4568, 205.8768)
  point P5 (148.307, 203.8496)
  point P6 (112.4082, 193.5106)
  point P7 (107.6247, 188.8434)
  point P8 (96.4049, 153.2101)
  point P9 (104.7984, 139.8337)
  point P10 (160.6075, 195.3173)
  point P11 (179.5109, 200.3088)
  point P12 (209.8152, 183.5009)
  point P13 (173.2694, 196.3001)
  point P14 (215.9918, 171.5026)
  point P15 (235.8927, 154.7714)
  point P16 (249.7399, 123.0723)
  point P17 (245.1719, 117.2601)
  point P18 (304.9678, 117.6838)
  point P19 (303.2716, 113.7945)
  point P20 (300.7153, 128.5141)
  point P21 (293.3402, 129.517)
  point P22 (300.2454, 111.9308)
  point P23 (272.473, 126.1655)
  point P24 (261.378, 128.1562)
  point P25 (282.6727, 100.1889)
  point P26 (255.6117, 88.5164)
  point P27 (232.9905, 61.7009)
  point P28 (242.9824, 104.7503)
  point P29 (245.9044, 96.7053)
  point P30 (102.9635, 127.267)
  point P31 (94.5348, 118.3814)
  point P32 (103.9684, 71.3012)
  point P33 (110.7671, 69.2897)
  point P34 (119.8576, 60.4211)
  point P35 (120.9633, 57.9394)
  point P36 (114.3412, 34.5652)
  point P37 (120.424, 18.0367)
  point P38 (121.4772, 45.2498)
  point P39 (204.1678, 48.5986)
  point P40 (125.7421, 12.9474)
  point P41 (102.4227, 30.1789)
  point P42 (108.5055, 13.6504)
  point P43 (92.4329, 32.3103)
  point P44 (75.4234, 14.8752)
  point P45 (82.0823, 115.8862)
  point P46 (78.7643, 116.5488)
  point P47 (71.3386, 105.504)
  point P48 (71.4598, 101.1593)
  point P49 (61.3321, 93.4965)
  point P50 (84.6881, 62.6277)
  point P51 (83.3424, 41.1789)
  point P52 (66.3329, 23.7438)
  point P53 (61.1161, 93.5151)
  point P54 (303.9033, 115.2529)
  point P55 (139.8047, 246.284)
  dimension "d460" = 6.35
  dimension "d461" = 6.35
  dimension "d462" = 6.35
  dimension "d463" = 6.35
  dimension "d464" = 6.35
  dimension "d465" = 6.35
  dimension "d466" = 6.35
  dimension "d467" = 6.35
  dimension "d468" = 6.35
  dimension "d469" = 6.35
  dimension "d470" = 6.35
  dimension "d471" = 6.35
  dimension "d472" = 6.35
  dimension "d473" = 6.35
  dimension "d474" = 6.35
  dimension "d475" = 6.35
  dimension "d476" = 6.35
  dimension "d477" = 6.35
  dimension "d478" = 6.35
  dimension "d479" = 4.7752
  dimension "d480" = 4.7752
  dimension "d481" = 4.7752
  dimension "d482" = 4.7752
  dimension "d483" = 6.35
  dimension "d484" = 6.35
  dimension "d485" = 6.35
  dimension "d486" = 6.35
  dimension "d487" = 4.7752
  dimension "d488" = 6.35
  dimension "d489" = 6.35
  dimension "d490" = 6.35
  dimension "d491" = 4.7752
  dimension "d492" = 4.7752
  dimension "d493" = 4.7752
  dimension "d494" = 6.35
  dimension "d495" = 6.35
  dimension "d496" = 6.35
  dimension "d497" = 4.7752
  dimension "d498" = 4.7752
  dimension "d499" = 4.7752
  dimension "d500" = 6.35
  dimension "d501" = 6.35
  dimension "d502" = 6.35
  dimension "d503" = 6.35
  dimension "d504" = 4.7752
  dimension "d505" = 4.7752
  dimension "d506" = 4.7752
  dimension "d507" = 6.35
  dimension "d508" = 6.35
  dimension "d509" = 6.35
  dimension "d510" = 4.7752
  dimension "d511" = 6.35
  dimension "d512" = 6.35
  dimension "d513" = 4.7752
  dimension "d514" = 4.7752
  dimension "d515" = 4.7752
  dimension "d516" = 6.35
  dimension "d517" = 6.35
  dimension "d518" = 6.35
  dimension "d519" = 4.7752
  dimension "d520" = 6.35
  dimension "d521" = 6.35
  dimension "d522" = 6.35
  dimension "d523" = 4.7752
  constraints: 317 point on circle, 154 end point, 145 tangent, 123 centre point, 114 point on line, 41 equal radius, 39 parallel, 20 concentric, 5 collinear, 2 midpoint, 91 other
  measures "d460" distance between parallel lines of L49 L58
  measures "d461" radial gap between concentric circles of A125 A166
  measures "d463" radial gap between concentric circles of A153 A168
  measures "d464" radial gap between concentric circles of A136 A169
  measures "d466" radial gap between concentric circles of A122 A171
  measures "d467" radial gap between concentric circles of A145 A172
  measures "d468" distance between parallel lines of L57 L66
  measures "d469" radial gap between concentric circles of A144 A177
  measures "d470" radial gap between concentric circles of A152 A178
  measures "d471" radial gap between concentric circles of A143 A179
  measures "d472" radial gap between concentric circles of A151 A180
  measures "d474" radial gap between concentric circles of A127 A182
  measures "d476" radial gap between concentric circles of A124 A184
  measures "d477" distance between parallel lines of L68 L90
  measures "d478" distance between parallel lines of L67 L91
  measures "d479" radius of A187
  measures "d480" radius of A189
  measures "d481" radius of A190
  measures "d482" diameter of A191
  measures "d483" distance between parallel lines of L67 L93
  measures "d484" distance between parallel lines of L70 L94
  measures "d485" distance between parallel lines of L71 L95
  measures "d486" distance between parallel lines of L69 L96
  measures "d487" radius of A196
  measures "d488" distance between parallel lines of L72 L97
  measures "d489" distance between parallel lines of L69 L98
  measures "d490" distance between parallel lines of L73 L99
  measures "d491" radius of A206
  measures "d492" radius of A209
  measures "d493" radius of A211
  measures "d494" distance between parallel lines of L73 L100
  measures "d495" distance between parallel lines of L74 L101
  measures "d496" distance between parallel lines of L81 L102
  measures "d497" radius of A215
  measures "d498" radius of A218
  measures "d499" radius of A220
  measures "d500" distance between parallel lines of L78 L104
  measures "d501" distance between parallel lines of L79 L105
  measures "d502" distance between parallel lines of L76 L106
  measures "d503" distance between parallel lines of L77 L107
  measures "d504" radius of A225
  measures "d505" radius of A229
  measures "d506" diameter of A231
  measures "d507" distance between parallel lines of L75 L108
  measures "d508" distance between parallel lines of L76 L109
  measures "d509" distance between parallel lines of L74 L110
  measures "d510" radius of A234
  measures "d511" distance between parallel lines of L77 L111
  measures "d512" distance between parallel lines of L80 L112
  measures "d513" radius of A240
  measures "d514" radius of A241
  measures "d515" radius of A244
  measures "d516" distance between parallel lines of L81 L115
  measures "d517" distance between parallel lines of L82 L116
  measures "d518" distance between parallel lines of L80 L117
  measures "d519" radius of A246
  measures "d520" distance between parallel lines of L71 L118
  measures "d521" distance between parallel lines of L87 L119
  measures "d522" distance between parallel lines of L83 L120
  measures "d523" radius of A252
extrude "Extrusion9" cut sketch "Sketch6" against normal blind 25.4 contours L90 A187 A186 A188 L91 A190 L92 A192 A185 A189 | A199 A194 A200 L96 A198 L95 A197 A193 A196 L94 A202 A195 A201 L93 | L97 A211 A204 A210 A205 A209 L99 A206 L98 A208 A203 A207 | L100 A218 A214 A219 A213 A220 L101 A216 A212 A217 L102 A215 | A227 A222 A228 L107 A229 L106 A230 A223 A232 L105 A225 A224 A226 | L108 A235 L109 A236 A233 A237 L110 A234 | L111 A244 L114 A238 L113 A241 L112 A240 A239 A242 | A247 A245 A248 L117 A249 L116 A246 L115 | L118 A254 L120 A255 A251 A256 L119 A253 A250 A252 | A257 L122 A258 L123 A259 L121 | A262 A260 A261 L125 A266 L126 A265 A263 A264 L124 | L127 A272 A269 A273 A268 A274 L128 A270 A267 A271 | L129 A279 L131 A278 A276 A277 L130 A275 | L132 A283 A281 A284 L133 A285 A280 L134 A282
body "Solid3"
